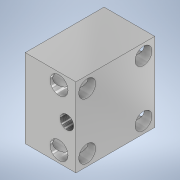
# Autodesk Inventor part: Acople de soporte de motor
Saved by Autodesk Inventor 2020 (Build 240168000, 168)
## iProperties
Created: 2020-05-15
Part Number: Acople de soporte de motor
Material: Aluminum 6061
Document SubType Name: Modeling
Designer: Dante
Density: 2.7 g/cm^3
Appearance: Aluminum - Dark
Mass: 450.818 g
Surface Area: 345.432 cm^2
Volume: 166.97 cm^3
Author: Dante
Autodesk Inventor part; units mm, degrees
ref_plane "YZ Plane" through (0, 0, 0) normal (1, 0, 0) x (0, 1, 0)
ref_plane "XZ Plane" through (0, 0, 0) normal (0, 1, 0) x (-1, 0, 0)
ref_plane "XY Plane" through (0, 0, 0) normal (0, 0, 1) x (1, 0, 0)
sketch "Sketch1" plane through (0, 0, 0) normal (0, 0, 1) x (1, 0, 0)
  line L0 (-45.5501, -290.4408) -> (-13.5501, -290.4408)
  circle A0 centre (-28.5501, -230.4408) radius 8
  line L1 (-45.5501, -220.4408) -> (-13.5501, -220.4408)
  circle A1 centre (-28.5501, -230.4408) radius 6
  line L2 (-13.5501, -290.4408) -> (-13.5501, -220.4408)
  circle A2 centre (-28.5501, -280.4408) radius 6
  circle A3 centre (-28.5501, -280.4408) radius 8
  circle A4 centre (-21.5501, -255.4408) radius 6
  line L3 (-36.5501, -280.4408) -> (-36.5501, -275.1231)
  line L4 (-50.5501, -255.4408) -> (-39.5501, -255.4408)
  line L5 (-45.5501, -290.4408) -> (-13.5501, -290.4408)
  circle A5 centre (-28.5501, -230.4408) radius 8
  line L6 (-45.5501, -220.4408) -> (-13.5501, -220.4408)
  circle A6 centre (-28.5501, -230.4408) radius 6
  line L7 (-13.5501, -290.4408) -> (-13.5501, -220.4408)
  circle A7 centre (-28.5501, -280.4408) radius 6
  circle A8 centre (-28.5501, -280.4408) radius 8
  circle A9 centre (-21.5501, -255.4408) radius 6
  line L8 (-36.5501, -280.4408) -> (-36.5501, -275.1231)
  line L9 (-50.5501, -255.4408) -> (-39.5501, -255.4408)
  line L10 (-58.5501, -290.4408) -> (-58.5501, -220.4408)
  line L11 (-58.5501, -290.4408) -> (-13.5501, -290.4408)
  circle A10 centre (-28.5501, -230.4408) radius 8
  line L12 (-58.5501, -220.4408) -> (-13.5501, -220.4408)
  circle A11 centre (-28.5501, -230.4408) radius 6
  line L13 (-13.5501, -290.4408) -> (-13.5501, -220.4408)
  circle A12 centre (-28.5501, -280.4408) radius 6
  circle A13 centre (-28.5501, -280.4408) radius 8
  circle A14 centre (-21.5501, -255.4408) radius 6
  line L14 (-36.5501, -280.4408) -> (-36.5501, -275.1231)
  line L15 (-58.5501, -255.4408) -> (-47.5501, -255.4408)
  line L16 (-49.5501, -286.9408) -> (-49.5501, -273.9408)
  line L17 (-40.5501, -280.4408) -> (-40.5501, -284.0729)
  line L18 (-49.5501, -273.9408) -> (-41.5501, -273.9408)
  line L19 (-41.5501, -273.9408) -> (-41.5501, -286.9408)
  line L20 (-41.5501, -286.9408) -> (-49.5501, -286.9408)
  line L21 (-49.5501, -223.9408) -> (-49.5501, -236.9408)
  line L22 (-49.5501, -236.9408) -> (-41.5501, -236.9408)
  line L23 (-41.5501, -236.9408) -> (-41.5501, -223.9408)
  line L24 (-41.5501, -223.9408) -> (-49.5501, -223.9408)
  line L25 (-15.5501, -255.4408) -> (-15.5501, -261.6781)
  circle A15 centre (-28.5501, -241.9408) radius 1.5
  circle A16 centre (-28.5501, -268.9408) radius 1.5
  point P0 (-13.5501, -220.4408)
  dimension "d11" = 16
  dimension "d33" = 16
  dimension "d55" = 16
  dimension "d58" = 12
  dimension "d5" = 16
  dimension "d6" = 10
  dimension "d7" = 12
  dimension "d9" = 15
  dimension "d10" = 12
  dimension "d12" = 10
  dimension "d13" = 15
  dimension "d14" = 12
  dimension "d15" = 8
  dimension "d27" = 16
  dimension "d28" = 10
  dimension "d29" = 12
  dimension "d31" = 15
  dimension "d32" = 12
  dimension "d34" = 10
  dimension "d35" = 15
  dimension "d36" = 12
  dimension "d37" = 8
  dimension "d49" = 16
  dimension "d51" = 12
  dimension "d52" = 45
  dimension "d53" = 15
  dimension "d54" = 12
  dimension "d56" = 10
  dimension "d57" = 15
  dimension "d59" = 8
  dimension "d95" = 8
  dimension "d96" = 36
  dimension "d115" = 1
  dimension "d116" = 13
  dimension "d121" = 3
  dimension "d122" = 11.5
  constraints: 52 end point, 13 centre point, 6 coincident, 5 symmetric about line, 4 horizontal alignment, 4 vertical, 2 perpendicular, 2 tangent, 1 midpoint, 9 other
  measures "d5" diameter of A0
  measures "d6" distance from line of L1 A0.centre
  measures "d7" diameter of A1
  measures "d9" distance from line of A0.centre L2
  measures "d10" diameter of A2
  measures "d12" distance from line of L0 A2.centre
  measures "d13" distance from line of A2.centre L2
  measures "d14" diameter of A4
  measures "d15" distance from line of A4.centre L2
  measures "d27" diameter of A5
  measures "d28" distance from line of L6 A5.centre
  measures "d29" diameter of A6
  measures "d31" distance from line of A5.centre L7
  measures "d32" diameter of A7
  measures "d34" distance from line of L5 A7.centre
  measures "d35" distance from line of A7.centre L7
  measures "d36" diameter of A9
  measures "d37" distance from line of A9.centre L7
  measures "d49" diameter of A10
  measures "d51" diameter of A11
  measures "d52" distance of L10.start L13.start
  measures "d53" distance from line of A10.centre L13
  measures "d54" diameter of A12
  measures "d56" distance from line of L11 A12.centre
  measures "d57" distance from line of A12.centre L13
  measures "d59" distance from line of point (-21.55, -255.441) L13
  measures "d95" distance of L16.end L18.end
  measures "d96" distance between parallel lines of L13 L16
  measures "d115" distance between parallel lines of L19 L17
  measures "d116" distance of L16.start L16.end
  measures "d121" diameter of A15
  measures "d122" distance of A15.centre A10.centre
ref_plane "Work Plane1" through (-18.5501, -290.4408, 0) normal (1, 0, 0) x (0, 0, -1)
extrude "Extrusion5" add sketch "Sketch1" along normal blind 70 contours L11 L10 L12 L1 L2 L0 | L16 L18 L19 L20 | L24 L23 L22 L21 | A15 | A16
sketch "Sketch3" plane through (-13.5501, -290.4408, 0) normal (1, 0, 0) x (0, 0, -1)
  circle A0 centre (-10, 10) radius 4
  line L0 (0, 0) -> (-70, 0) projected
  circle A1 centre (-60, 10) radius 4
  line L1 (0, 0) -> (0, 70) projected
  circle A2 centre (-10, 10) radius 7.5
  circle A3 centre (-60, 10) radius 7.5
  circle A4 centre (-10, 60) radius 4
  line L2 (0, 70) -> (-70, 70)
  circle A5 centre (-60, 60) radius 4
  line L3 (0, 70) -> (0, 0)
  circle A6 centre (-10, 60) radius 7.5
  circle A7 centre (-60, 60) radius 7.5
  dimension "d102" = 8
  dimension "d103" = 10
  dimension "d105" = 8
  dimension "d106" = 50
  dimension "d107" = 10
  dimension "d108" = 10
  dimension "d109" = 15
  dimension "d110" = 15
  dimension "d117" = 15
  dimension "d118" = 15
  constraints: 8 centre point, 4 coincident, 4 end point
  measures "d102" diameter of A0
  measures "d103" distance from line of A0.centre L0
  measures "d105" diameter of A1
  measures "d106" distance of A1.centre A0.centre
  measures "d107" distance from line of L1 A0.centre
  measures "d108" distance from line of L0 A1.centre
  measures "d109" diameter of A2
  measures "d110" diameter of A3
  measures "d117" diameter of A6
  measures "d118" diameter of A7
extrude "Extrusion7" cut sketch "Sketch3" against normal blind 100 contours A0 | A1 | A4 | A5
extrude "Extrusion8" cut sketch "Sketch3" against normal blind 36
thread "Thread1" size "M12x1.5" class "6H" standard "ISO Metric profile" length 348
extrude "Extrusion9" cut sketch "Sketch1" along normal blind 6 contours A15 | A16
body "Solid2"
